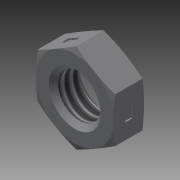
# Autodesk Inventor part: 2LOPRO-NUT
Saved by Autodesk Inventor 2014 SP2 (Build 180246200, 246)
## iProperties
Created: 2018-12-09
Part Number: 2LOPRO-NUT
Material: Generic
Catalog Web Link: www.cadenas.de
Description: 2 Series LoPro Nut-Capacitiy up to 210 lbs Each
Vendor: COLSONGROUP
Document SubType Name: Modeling
Designer: psadmin
Manufacturer: COLSONGROUP
Mass: 0.686906 g
Surface Area: 6.41313 cm^2
Volume: 0.686906 cm^3
Density: 1 g/cm^3
Appearance: PSOLRGB-175-175-175
Category: PARTsolutions
Company: COLSONGROUP
Title: 2LOPRO-NUT
Author: Cadenas PARTsolutions
Comments: Capacitiy up to 210 lbs Each
PSOL_IDENT_0: {$CADENAS_DATA\23d-libs\colsongroup\colson\casters\2_series_lopro\2_series_lopro_nut.prj},172 {VTYP=
PSOL_IDENT_1: 3D},{NB=2LOPRO-NUT},{LINA=2LOPRO-NUT},{NN=2 Series LoPro Nut},{DATE=13.07.2017 07:15:58},{GEOMDATE=3
PSOL_IDENT_2: 0.01.2017 12:40:00},{VERSION=},{LINEID=40},{WBVAR=},{WBNUMERIC=}  {NB=2LOPRO-NUT},{LINA=2LOPRO-NUT},
PSOL_IDENT_3: {KT=DUMMY},{PN=2LOPRO-NUT}
NN: 2 Series LoPro Nut
NT: Capacitiy up to 210 lbs Each
NB: 2LOPRO-NUT
NBSYN: $PN.
LINA: 2LOPRO-NUT
PN: 2LOPRO-NUT
SUPPLIER: COLSONGROUP
ARTICLENO: 2LOPRO-NUT
BOMINFO: 2LOPRO-NUT
CREATOR: CADENAS GmbH
Autodesk Inventor part; units mm, degrees
sketch "Sketch_1" plane through (0, 0, 0) normal (1, 0, 0) x (0, 1, 0)
  line L0 (0, -5.588) -> (0, 0)
  line L1 (4.7625, 0) -> (3.9027, -0.8598)
  line L2 (3.9027, -0.8598) -> (3.9027, -4.7282)
  line L3 (3.9027, -4.7282) -> (4.7625, -5.588)
  line L4 (4.7625, -5.588) -> (7.112, -5.588)
  line L5 (7.112, -5.588) -> (8.5344, -5.2069)
  line L6 (8.5344, -5.2069) -> (8.5344, -0.3811)
  line L7 (8.5344, -0.3811) -> (7.112, 0)
  line L8 (7.112, 0) -> (4.7625, 0)
  constraints: 18 end point
revolve "Revolution1" add sketch "Sketch_1" angle 360 about axis through (0, 0, -5.588) along (0, 0, -1)
thread "Thread1" size "3/8-16 UNC" class "2B" standard "ANSI Unified Screw Threads" full length
sketch "Sketch_2" plane through (0, 0, 0) normal (0, 0, 1) x (1, 0, 0)
  circle A0 centre (0, 0) radius 15.24
  line L0 (-7.112, -4.1061) -> (0, -8.2122)
  line L1 (0, -8.2122) -> (7.112, -4.1061)
  line L2 (7.112, -4.1061) -> (7.112, 4.1061)
  line L3 (7.112, 4.1061) -> (0, 8.2122)
  line L4 (0, 8.2122) -> (-7.112, 4.1061)
  line L5 (-7.112, 4.1061) -> (-7.112, -4.1061)
  constraints: 12 end point, 1 centre point
extrude "Extrusion1" cut sketch "Sketch_2" against normal blind 5.588
sketch "Sketch_3" plane through (7.112, 0, 0) normal (1, 0, 0) x (0, 0, -1)
  line L0 (2.159, 1.27) -> (2.159, -1.27)
  line L1 (2.159, -1.27) -> (3.429, -1.27)
  line L2 (3.429, -1.27) -> (3.429, 1.27)
  line L3 (3.429, 1.27) -> (2.159, 1.27)
  constraints: 8 end point
extrude "Extrusion2" cut sketch "Sketch_3" along normal mid plane 0.508
sketch "Sketch_4" plane through (-3.556, 6.1592, 0) normal (0.5, -0.866, 0) x (0, 0, -1)
  line L0 (2.159, 1.27) -> (2.159, -1.27)
  line L1 (2.159, -1.27) -> (3.429, -1.27)
  line L2 (3.429, -1.27) -> (3.429, 1.27)
  line L3 (3.429, 1.27) -> (2.159, 1.27)
  constraints: 8 end point
extrude "Extrusion3" cut sketch "Sketch_4" along normal mid plane 0.508
sketch "Sketch_5" plane through (-3.556, -6.1592, 0) normal (0.5, 0.866, 0) x (0, 0, -1)
  line L0 (2.159, 1.27) -> (2.159, -1.27)
  line L1 (2.159, -1.27) -> (3.429, -1.27)
  line L2 (3.429, -1.27) -> (3.429, 1.27)
  line L3 (3.429, 1.27) -> (2.159, 1.27)
  constraints: 8 end point
extrude "Extrusion4" cut sketch "Sketch_5" along normal mid plane 0.508
ref_plane "nut_XY" through (0, 0, 0) normal (0, 0, -1) x (1, 0, 0)
ref_plane "nut_YZ" through (0, 0, 0) normal (1, 0, 0) x (0, -1, 0)
ref_plane "nut_ZX" through (0, 0, 0) normal (0, -1, 0) x (0, 0, -1)
body "Solid1"
